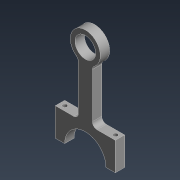
# Autodesk Inventor part: P012-Corps_bielle
Saved by Autodesk Inventor 2021.3 (Build 253353000, 353)
## iProperties
Created: 2022-03-31
Part Number: P012-Corps_bielle
Material: Générique
Document SubType Name: Modeling
Designer: remi
Density: 1 g/cm^3
Appearance: Par défaut
Author: remi
Autodesk Inventor part; units mm, degrees
ref_plane "YZ Plane" through (0, 0, 0) normal (1, 0, 0) x (0, 1, 0)
ref_plane "XZ Plane" through (0, 0, 0) normal (0, 1, 0) x (-1, 0, 0)
ref_plane "XY Plane" through (0, 0, 0) normal (0, 0, 1) x (1, 0, 0)
sketch "Sketch2" plane through (0, 0, 0) normal (0, 1, 0) x (-1, 0, 0)
  line L0 (0, -23.2) -> (0, 139.2) construction
  circle A0 centre (0, 100) radius 11
  arc A1 (7.5, 85.8667) -> (-7.5, 85.8667) centre (0, 100) ccw
  line L1 (-7.5, 85.8667) -> (-7.5, 30)
  line L2 (-7.5, 30) -> (-32, 30)
  line L3 (-32, 30) -> (-32, 0)
  line L4 (-32, 0) -> (-22, 0)
  arc A2 (22, 0) -> (-22, 0) centre (0, 0) ccw
  line L5 (22, 0) -> (32, 0)
  line L6 (32, 0) -> (32, 30)
  line L7 (32, 30) -> (7.5, 30)
  line L8 (7.5, 30) -> (7.5, 85.8667)
  dimension "d0" = 15
  dimension "d2" = 10
  dimension "d3" = 22
  dimension "d4" = 30
  dimension "d5" = 100
  dimension "d7" = 5
  dimension "d8" = 22
  constraints: 16 end point, 6 perpendicular, 4 equal length, 4 point on circle, 3 centre point, 1 coincident, 1 horizontal, 1 horizontal alignment, 1 point on line, 1 vertical
  measures "d0" distance between parallel lines of L1 L8
  measures "d2" distance of L3.end L4.end
  measures "d3" radius of A2
  measures "d4" distance of L2.end L3.end
  measures "d5" distance of A0.centre A2.centre
  measures "d7" radial gap between concentric circles of A0 A1
  measures "d8" diameter of A0
extrude "Extrusion1" add sketch "Sketch2" along normal blind 10
fillet "Fillet1" radius 5 4 edges at (-7.5, 5, 30) (7.5, 5, 30) (7.5, 5, 85.8667) (-7.5, 5, 85.8667)
sketch "Sketch3" plane through (0, 0, 0) normal (0, 0, 1) x (1, 0, 0)
  line L0 (-22, 0) -> (-32, 0) construction
  line L1 (-32, 0) -> (-32, 10) construction
  line L2 (-22, 10) -> (-32, 10) construction
  line L3 (-22, 0) -> (-22, 10) construction
  line L4 (32, 0) -> (22, 0) construction
  line L5 (22, 0) -> (22, 10) construction
  line L6 (32, 10) -> (22, 10) construction
  line L7 (32, 0) -> (32, 10) construction
  line L8 (-32, 0) -> (-22, 10) construction
  line L9 (-22, 0) -> (-32, 10) construction
  line L10 (22, 0) -> (32, 10) construction
  line L11 (32, 0) -> (22, 10) construction
  point P0 (0, 0)
  point P1 (-27, 5)
  point P2 (27, 5)
  constraints: 8 end point, 3 perpendicular, 2 midpoint
hole "Hole1" at (-27, 5, 0) at (27, 5, 0) direction (0, 0, 1) diameter 4.5 end through all clearance for "Flat Head Machine Screw" size "M4" standard "Ansi Metric M Profile"
body "Solid1"
